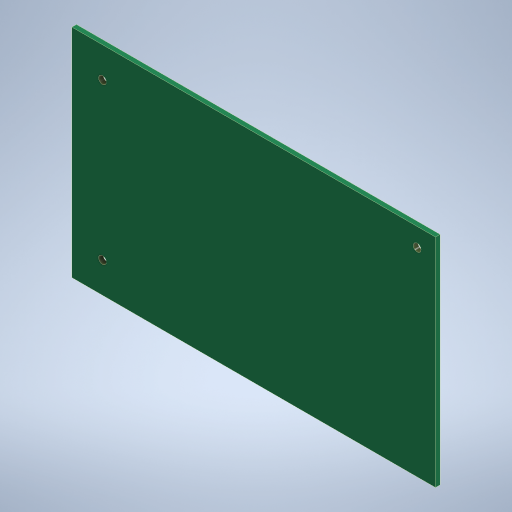
# Autodesk Inventor part: PCB
Saved by Autodesk Inventor 2023 (Build 270158000, 158)
## iProperties
Created: 2022-12-30
Part Number: PCB
Material: Generico
Document SubType Name: Modeling
Designer: Gabriele
Density: 1 g/cm^3
Appearance: Oliva scuro
Author: Gabriele
Autodesk Inventor part; units mm, degrees
ref_plane "YZ Plane" through (0, 0, 0) normal (1, 0, 0) x (0, 1, 0)
ref_plane "XZ Plane" through (0, 0, 0) normal (0, 1, 0) x (-1, 0, 0)
ref_plane "XY Plane" through (0, 0, 0) normal (0, 0, 1) x (1, 0, 0)
sketch "Schizzo1" plane through (0, 0, 0) normal (0, 0, 1) x (1, 0, 0)
  line L0 (-59.5, -35.5) -> (59.5, -35.5)
  line L1 (59.5, -35.5) -> (59.5, 35.5)
  line L2 (59.5, 35.5) -> (-59.5, 35.5)
  line L3 (-59.5, 35.5) -> (-59.5, -35.5)
  line L4 (-59.5, -35.5) -> (59.5, 35.5) construction
  line L5 (59.5, -35.5) -> (-59.5, 35.5) construction
  point P0 (0, 0)
  dimension "d0" = 119
  dimension "d1" = 71
  constraints: 12 end point, 2 midpoint, 2 parallel, 1 horizontal, 1 perpendicular
  measures "d0" distance of L1.end L2.end
  measures "d1" distance of L0.end L1.end
extrude "Estrusione1" add sketch "Schizzo1" along normal blind 1.5
sketch "Schizzo4" plane through (0, 0, 1.5) normal (0, 0, 1) x (1, 0, 0)
  line L0 (59.5, 35.5) -> (-59.5, 35.5) projected
  line L1 (59.5, -35.5) -> (59.5, 35.5) projected
  line L2 (-59.5, -35.5) -> (59.5, -35.5) projected
  circle A0 centre (-49.5, 25.5) radius 1.25
  circle A1 centre (-49.5, -25.5) radius 1.25
  line L3 (-59.5, 35.5) -> (-59.5, -35.5) projected
  circle A2 centre (53.5, 29.5) radius 1.25
  point P0 (0, 0)
  dimension "d17" = 2.5
  dimension "d18" = 2.5
  dimension "d19" = 10
  dimension "d20" = 10
  dimension "d21" = 10
  dimension "d22" = 10
  dimension "d24" = 2.5
  dimension "d27" = 6
  dimension "d28" = 6
  constraints: 3 centre point
  measures "d17" diameter of A0
  measures "d18" diameter of A1
  measures "d19" distance from line of L0 A0.centre
  measures "d20" distance from line of L3 A0.centre
  measures "d21" distance from line of L2 A1.centre
  measures "d22" distance from line of L3 A1.centre
  measures "d24" diameter of A2
  measures "d27" distance from line of L0 A2.centre
  measures "d28" distance from line of L1 A2.centre
extrude "Estrusione3" cut sketch "Schizzo4" against normal blind 1.5 contours A0 | A1 | A2
